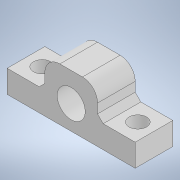
# Autodesk Inventor part: Modular_Single_Axle_V41Y
Saved by Autodesk Inventor 2021 (Build 250183000, 183)
## iProperties
Created: 2021-06-07
Part Number: Modular_Single_Axle_V41Y
Material: Generic
Document SubType Name: Modeling
Designer: Work
Density: 1 g/cm^3
Appearance: Default
Author: Work
Autodesk Inventor part; units mm, degrees
ref_plane "YZ Plane" through (0, 0, 0) normal (1, 0, 0) x (0, 1, 0)
ref_plane "XZ Plane" through (0, 0, 0) normal (0, 1, 0) x (-1, 0, 0)
ref_plane "XY Plane" through (0, 0, 0) normal (0, 0, 1) x (1, 0, 0)
sketch "Sketch1" plane through (0, 0, 0) normal (0, 1, 0) x (-1, 0, 0)
  line L0 (0, 0) -> (34, 0)
  line L1 (34, 0) -> (34, -10)
  line L2 (34, -10) -> (0, -10)
  line L3 (0, -10) -> (0, 0)
  dimension "d0" = 34
  dimension "d1" = 10
  constraints: 8 end point, 2 parallel, 1 horizontal, 1 perpendicular
  measures "d0" distance of L1.end L2.end
  measures "d1" distance of L1.end L0.end
extrude "Extrusion1" add sketch "Sketch1" along normal blind 6
sketch "Sketch3" plane through (0, 6, 0) normal (0, 1, 0) x (1, 0, 0)
  circle A0 centre (-4.3, 5) radius 2.325
  line L0 (0, 10) -> (-34, 10) projected
  circle A1 centre (-29.7, 5) radius 2.325
  line L1 (-34, 10) -> (-34, 0) projected
  line L2 (0, 0) -> (0, 10) projected
  dimension "d4" = 4.65
  dimension "d5" = 5
  dimension "d6" = 4.65
  dimension "d7" = 5
  dimension "d9" = 4.3
  dimension "d10" = 4.3
  constraints: 2 centre point
  measures "d4" diameter of A0
  measures "d5" distance from line of L0 A0.centre
  measures "d6" diameter of A1
  measures "d7" distance from line of L0 A1.centre
  measures "d9" distance from line of L1 A1.centre
  measures "d10" distance from line of L2 A0.centre
extrude "Extrusion2" cut sketch "Sketch3" against normal through all
sketch "Sketch4" plane through (0, 6, 0) normal (0, 1, 0) x (1, 0, 0)
  line L0 (-34, 0) -> (0, 0) projected
  line L1 (0, 10) -> (-34, 10) projected
  line L2 (-10, 0) -> (-24, 0)
  line L3 (-24, 0) -> (-24, 10)
  line L4 (-24, 10) -> (-10, 10)
  line L5 (-10, 10) -> (-10, 0)
  circle A0 centre (-4.3, 5) radius 2.325 projected
  line L6 (-34, 10) -> (-34, 0) projected
  line L7 (0, 0) -> (0, 10) projected
  point P0 (-10, 10)
  point P1 (-24, 0)
  dimension "d34" = 14
  dimension "d35" = 10
  constraints: 8 end point, 2 parallel, 2 point on line, 1 horizontal, 1 perpendicular
  measures "d34" distance of L4.end L3.end
  measures "d35" distance between parallel lines of L6 L3
extrude "Extrusion3" add sketch "Sketch4" along normal blind 8 contours L3 L1 L5 L0
sketch "Sketch6" plane through (0, 0, -10) normal (0, 0, -1) x (-1, 0, 0)
  circle A0 centre (17, 6.38) radius 3.725
  line L0 (10, 14) -> (24, 14) projected
  line L1 (24, 6) -> (24, 14) projected
  point P0 (0, 0)
  dimension "d26" = 7.45
  dimension "d36" = 7.62
  dimension "d37" = 7
  constraints: 1 centre point
  measures "d26" diameter of A0
  measures "d36" distance from line of A0.centre L0
  measures "d37" distance from line of L1 A0.centre
extrude "Extrusion4" cut sketch "Sketch6" against normal through all
fillet "Fillet2" radius 4 2 edges at (-24, 14, -5) (-10, 14, -5)
chamfer "Chamfer1" distance 1.5 angle 45 2 edges at (-10, 6, -5) (-24, 6, -5)
body "Solid1"
